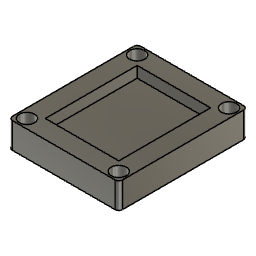
case v3 (Autodesk Fusion 360 design; units mm, degrees)
Autodesk Fusion 360 part; units mm, degrees
sketch "スケッチ1" plane through (0, 0, 0) normal (0, 0, 1) x (1, 0, 0)
  line L0 (0, 0) -> (30, 0)
  line L1 (30, 0) -> (30, 35)
  line L2 (30, 35) -> (0, 35)
  line L3 (0, 35) -> (0, 0)
  dimension "d1" = 35
  dimension "d2" = 30
  constraint horizontal L0
  constraint vertical L1
  constraint horizontal L2
  constraint vertical L3
  constraint coincident L0.start L3.end
  measures "d1" distance of L0.end L1.end
  measures "d2" distance of L0.start L0.end
extrude "押し出し1" add sketch "スケッチ1" along normal blind 7
sketch "スケッチ2" plane through (0, 0, 7) normal (0, 0, 1) x (-1, 0, 0)
  line L0 (0, -35) -> (0, 0)
  line L1 (0, 0) -> (-30, 0)
  line L2 (-30, 0) -> (-30, -35)
  line L3 (-30, -35) -> (0, -35)
  line L4 (-5, -30) -> (-25, -30)
  line L5 (-25, -30) -> (-25, -5)
  line L6 (-25, -5) -> (-5, -5)
  line L7 (-5, -5) -> (-5, -30)
  dimension "d5" = 20
  dimension "d6" = 25
  constraint horizontal L4
  constraint vertical L5
  constraint horizontal L6
  constraint vertical L7
  measures "d5" distance of L4.start L4.end
  measures "d6" distance of L4.end L5.end
extrude "押し出し2" cut sketch "スケッチ2" against normal blind 3 contours L4 L5 L6 L7
fillet "フィレット1" radius 1 4 edges at (30, 0, 3.5) (30, 35, 3.5) (0, 0, 3.5) (0, 35, 3.5)
sketch "スケッチ3" plane through (0, 0, 7) normal (0, 0, 1) x (-1, 0, 0)
  arc A0 (-1, -35) -> (0, -34) centre (-1, -34) ccw
  line L0 (0, -34) -> (0, -1)
  arc A1 (0, -1) -> (-1, 0) centre (-1, -1) ccw
  line L1 (-1, 0) -> (-29, 0)
  arc A2 (-29, 0) -> (-30, -1) centre (-29, -1) ccw
  line L2 (-30, -1) -> (-30, -34)
  arc A3 (-30, -34) -> (-29, -35) centre (-29, -34) ccw
  line L3 (-29, -35) -> (-1, -35)
  line L4 (-25, -30) -> (-25, -5)
  line L5 (-25, -5) -> (-5, -5)
  line L6 (-5, -5) -> (-5, -30)
  line L7 (-5, -30) -> (-25, -30)
  circle A4 centre (-27.5, -2.5) radius 2.05
  circle A5 centre (-2.5, -2.5) radius 2.05
  circle A6 centre (-2.5, -32.5) radius 2.05
  circle A7 centre (-27.5, -32.5) radius 2.05
  dimension "d17" = 4.1
  dimension "d18" = 4.1
  dimension "d19" = 4.1
  dimension "d20" = 4.1
  measures "d17" diameter of A4
  measures "d18" diameter of A5
  measures "d19" diameter of A6
  measures "d20" diameter of A7
extrude "押し出し3" cut sketch "スケッチ3" against normal blind 7 contours A4 | A5 | A6 | A7
